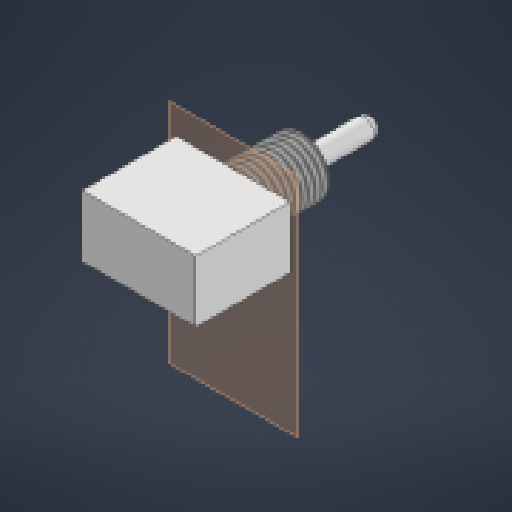
# Autodesk Inventor part: AST13SEBQ
Saved by Autodesk Inventor 2024 (Build 280153000, 153)
## iProperties
Created: 2026-08-20
Part Number: AST13SEBQ
Material: Generic
Document SubType Name: Modeling
Designer: schar
Density: 1 g/cm^3
Appearance: Default
Author: schar
Autodesk Inventor part; units mm, degrees
ref_plane "YZ Plane" through (0, 0, 0) normal (1, 0, 0) x (0, 1, 0)
ref_plane "XZ Plane" through (0, 0, 0) normal (0, 1, 0) x (-1, 0, 0)
ref_plane "XY Plane" through (0, 0, 0) normal (0, 0, 1) x (1, 0, 0)
ref_plane "Work Plane1" through (0, 0, 0) normal (0, 0, 1) x (1, 0, 0)
sketch "Sketch1" plane through (0, 0, 0) normal (0, 0, 1) x (1, 0, 0)
  arc A0 (-4.3529, 18.17) -> (-4.3529, 17.33) centre (-7.5, 17.75) ccw projected
  circle A1 centre (-7.5, 17.75) radius 3.175
  point P0 (0, 0)
  dimension "d0" = 6.35
  constraints: 1 centre point, 1 coincident
  measures "d0" diameter of A1
extrude "Extrusion1" add sketch "Sketch1" against normal blind 7.58
sketch "Sketch2" plane through (-7.5, 17.75, 0) normal (0, 0, 1) x (1, 0, 0)
  line L0 (-6.35, -3.425) -> (6.35, -3.425)
  line L1 (6.35, -3.425) -> (6.35, 3.425)
  line L2 (6.35, 3.425) -> (-6.35, 3.425)
  line L3 (-6.35, 3.425) -> (-6.35, -3.425)
  line L4 (-6.35, -3.425) -> (6.35, 3.425) construction
  line L5 (6.35, -3.425) -> (-6.35, 3.425) construction
  point P0 (7.5, -17.75)
  point P1 (0, 0)
  dimension "d3" = 12.7
  dimension "d4" = 6.85
  constraints: 12 end point, 2 midpoint, 2 parallel, 1 horizontal, 1 perpendicular
  measures "d3" distance of L2.end L1.end
  measures "d4" distance of L1.end L0.end
extrude "Extrusion2" add sketch "Sketch2" along normal blind 10.5
sketch "Sketch3" plane through (-7.5, 17.75, -7.58) normal (0, 0, -1) x (-1, 0, 0)
  circle A0 centre (0, 0) radius 2.6
  point P0 (-7.5, -17.75)
  dimension "d7" = 5.2
  constraints: 1 centre point
  measures "d7" diameter of A0
extrude "Extrusion3" cut sketch "Sketch3" against normal blind 4
sketch "Sketch4" plane through (-7.5, 17.75, -3.58) normal (0, 0, -1) x (-1, 0, 0)
  circle A0 centre (0, 0) radius 1.1094
  point P0 (-7.5, -17.75)
  constraints: 1 centre point
extrude "Extrusion4" add sketch "Sketch4" along normal blind 12
fillet "Fillet1" radius 1 1 edges at (-6.3906, 17.75, -15.58)
thread "Thread1" size "M7x0.75" class "6g" standard "ISO Metric profile" length 15.103
chamfer "Chamfer1" distance 1 angle 45 1 edges at (-4.9, 17.75, -3.58)
body "Solid1"
